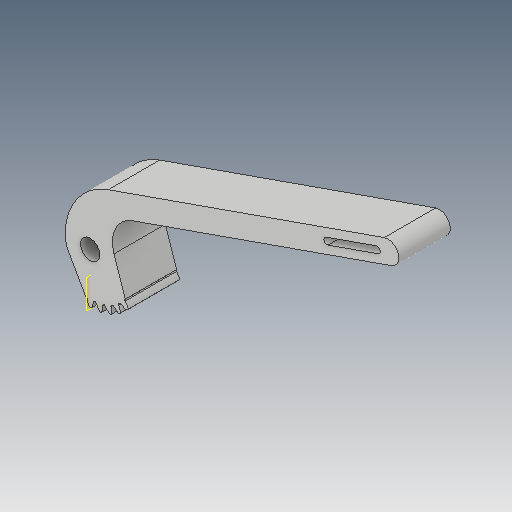
# Autodesk Inventor part: GripperLever_right_v2
Saved by Autodesk Inventor 2021.4 (Build 254397000, 397)
## iProperties
Created: 2022-04-22
Part Number: GripperLever_right_v2
Material: Generisch
Document SubType Name: Modeling
Designer: ALEX
Density: 1 g/cm^3
Appearance: Vorgabe
Mass: 2.14973 g
Surface Area: 19.5452 cm^2
Volume: 2.14973 cm^3
Di: 13,833 mm
GearThickness: 9,000 mm
Lever_Do: 8,000 mm
d: 15,000 mm
Author: ALEX
Autodesk Inventor part; units mm, degrees
ref_plane "YZ Plane" through (0, 0, 0) normal (1, 0, 0) x (0, 1, 0)
ref_plane "XZ Plane" through (0, 0, 0) normal (0, 1, 0) x (-1, 0, 0)
ref_plane "XY Plane" through (0, 0, 0) normal (0, 0, 1) x (1, 0, 0)
sketch "Skizze1" plane through (0, 0, 0) normal (0, 0, 1) x (1, 0, 0)
  circle A0 centre (0, 0) radius 6.9167 construction
  circle A1 centre (0, 0) radius 8 construction
  arc A2 (-0.4858, -7.0515) -> (-0.6563, -6.8855) centre (-0.6743, -7.0746) ccw
  arc A3 (-0.4858, -7.0515) -> (-0.1749, -7.9981) centre (2.0604, -6.7398) ccw
  line L0 (0, 0) -> (0.8362, -7.9562) construction
  line L1 (0, 0) -> (0, -8) construction
  arc A4 (-0.1749, -7.9981) -> (0.1749, -7.9981) centre (0, 0) ccw
  arc A5 (0.1749, -7.9981) -> (0.4858, -7.0515) centre (-2.0604, -6.7398) ccw
  arc A6 (0.6563, -6.8855) -> (0.4858, -7.0515) centre (0.6743, -7.0746) ccw
  arc A7 (0.6563, -6.8855) -> (0.723, -6.8788) centre (0, 0) ccw
  line L2 (0, 0) -> (0, -8) construction
  circle A8 centre (0, 0) radius 7.5 construction
  circle A9 centre (0, 0) radius 4
  circle A10 centre (0, 0) radius 1.55
  circle A11 centre (0, 0) radius 7.0477 construction
  line L3 (-0.3927, -7.4897) -> (2.0604, -6.7398) construction
  line L4 (0.3927, -7.4897) -> (-2.0604, -6.7398) construction
  line L5 (0, 0) -> (-0.723, -6.8788) construction
  arc A12 (-0.723, -6.8788) -> (-0.6563, -6.8855) centre (0, 0) ccw
  arc A13 (2.0735, -6.5985) -> (2.1374, -6.5781) centre (0, 0) ccw
  arc A14 (2.0735, -6.5985) -> (1.9412, -6.7964) centre (2.1305, -6.7798) ccw
  arc A15 (1.834, -7.7869) -> (1.9412, -6.7964) centre (-0.6141, -7.0209) ccw
  arc A16 (0.723, -6.8788) -> (0.7896, -6.8714) centre (0, 0) ccw
  arc A17 (1.4918, -7.8597) -> (1.834, -7.7869) centre (0, 0) ccw
  arc A18 (0.991, -6.9984) -> (0.7896, -6.8714) centre (0.8113, -7.0602) ccw
  arc A19 (0.991, -6.9984) -> (1.4918, -7.8597) centre (3.4166, -6.1641) ccw
  arc A20 (3.4001, -6.0232) -> (3.4583, -5.99) centre (0, 0) ccw
  arc A21 (3.4001, -6.0232) -> (3.3119, -6.2443) centre (3.4935, -6.1887) ccw
  arc A22 (3.4129, -7.2355) -> (3.3119, -6.2443) centre (0.8591, -6.9951) ccw
  arc A23 (2.1374, -6.5781) -> (2.201, -6.5571) centre (0, 0) ccw
  arc A24 (3.0933, -7.3778) -> (3.4129, -7.2355) centre (0, 0) ccw
  arc A25 (2.4243, -6.6395) -> (2.201, -6.5571) centre (2.2615, -6.7373) ccw
  arc A26 (2.4243, -6.6395) -> (3.0933, -7.3778) centre (4.6236, -5.3191) ccw
  arc A27 (4.5781, -5.1847) -> (4.6282, -5.1401) centre (0, 0) ccw
  arc A28 (4.5781, -5.1847) -> (4.5378, -5.4193) centre (4.7039, -5.3271) ccw
  arc A29 (4.8427, -6.3678) -> (4.5378, -5.4193) centre (2.2947, -6.6637) ccw
  arc A30 (3.4583, -5.99) -> (3.5162, -5.9562) centre (0, 0) ccw
  arc A31 (4.5596, -6.5734) -> (4.8427, -6.3678) centre (0, 0) ccw
  arc A32 (3.7518, -5.9903) -> (3.5162, -5.9562) centre (3.6128, -6.1198) ccw
  arc A33 (3.7518, -5.9903) -> (4.5596, -6.5734) centre (5.6284, -4.2415) ccw
  arc A34 (5.5561, -4.1195) -> (5.5957, -4.0655) centre (0, 0) ccw
  arc A35 (5.5561, -4.1195) -> (5.5653, -4.3574) centre (5.7087, -4.2327) ccw
  arc A36 (6.0608, -5.2218) -> (5.5653, -4.3574) centre (3.63, -6.041) ccw
  arc A37 (4.6282, -5.1401) -> (4.6777, -5.095) centre (0, 0) ccw
  arc A38 (5.8267, -5.4818) -> (6.0608, -5.2218) centre (0, 0) ccw
  arc A39 (4.9153, -5.0794) -> (4.6777, -5.095) centre (4.8062, -5.235) ccw
  arc A40 (4.9153, -5.0794) -> (5.8267, -5.4818) centre (6.3873, -2.9786) ccw
  line L6 (-0.723, -6.8788) -> (-3.4872, -1.9595)
  line L7 (5.5957, -4.0655) -> (3.7896, 1.2803)
  point P0 (2.4721, -7.6085)
  point P1 (1.9413, -7.2444)
  point P2 (1.6633, -7.8252)
  point P3 (1.6633, -7.8252)
  point P4 (1.1731, -7.4077)
  point P5 (4, -6.9282)
  point P6 (3.4051, -6.6825)
  point P7 (3.2539, -7.3084)
  point P8 (3.2539, -7.3084)
  point P9 (2.6876, -7.0019)
  point P10 (5.353, -5.9452)
  point P11 (4.72, -5.8285)
  point P12 (4.7023, -6.4721)
  point P13 (4.7023, -6.4721)
  point P14 (4.0846, -6.2901)
  point P15 (6.4721, -4.7023)
  point P16 (5.8287, -4.7198)
  point P17 (5.9452, -5.353)
  point P18 (5.9452, -5.353)
  point P19 (5.3032, -5.3034)
  point P20 (0.723, -6.8788)
  point P21 (2.1374, -6.5781)
  point P22 (3.4583, -5.99)
  point P23 (4.6282, -5.1401)
  point P24 (5.5957, -4.0655)
  dimension "d0" = 13.8333
  dimension "d1" = 16
  dimension "d2" = 0.19
  dimension "d6" = 0
  dimension "d9" = 15
  dimension "d10" = 0.7854
  dimension "Lever_Do" = 8
  dimension "d17" = 3.1
  dimension "d26" = 14.0954
  dimension "d74" = 12
  dimension "d75" = 6
  dimension "beta_circ" = 48
  constraints: 94 point on circle, 41 centre point, 16 end point, 8 coincident, 8 tangent, 3 concentric, 2 equal radius, 1 point on line, 1 vertical, 109 other
  measures "d0" diameter of A0
  measures "d1" diameter of A1
  measures "d2" radius of A2
  measures "d6" distance between parallel lines of L1 L2
  measures "d9" diameter of A8
  measures "d10" distance of L4.start L3.start
  measures "Lever_Do" diameter of A9
  measures "d17" diameter of A10
  measures "d26" diameter of A11
  measures "d74" angle of L0 L5
  measures "d75" angle of L5 L2
extrude "Extrusion1" add sketch "Skizze1" along normal blind 9
sketch "Skizze2" plane through (0, 0, 9) normal (0, 0, 1) x (1, 0, 0)
  line L0 (0, 0) -> (49.154, 0) construction
  arc A0 (3.7896, 1.2803) -> (-3.4872, -1.9595) centre (0, 0) ccw projected
  line L1 (48.5762, 25.6793) -> (49.7318, 22.3756)
  line L2 (49.3026, 23.6027) -> (2.1068, 7.0935) construction
  line L3 (0, 0) -> (1.1388, 3.8345) construction
  line L4 (49.154, 0) -> (49.154, 24.0275) construction
  circle A1 centre (0, 0) radius 4 construction
  line L5 (6.7484, 7.3399) -> (49.7318, 22.3756)
  line L6 (48.5762, 25.6793) -> (2.8793, 9.6944)
  circle A2 centre (0, 0) radius 8 construction
  arc A3 (2.8793, 9.6944) -> (-4, 0) centre (6.2704, 0) ccw
  arc A4 (6.7484, 7.3399) -> (3.7896, 1.2803) centre (8.3313, 2.8148) ccw
  circle A5 centre (0, 0) radius 1.55 projected
  line L7 (0, 0) -> (49.154, 17.1942) construction
  dimension "d39" = 19.28
  dimension "d70" = 8
  dimension "d72" = 50
  dimension "d96" = 6
  dimension "d97" = 1.3
  dimension "d98" = 3.5
  constraints: 16 end point, 6 point on circle, 5 point on line, 4 tangent, 3 centre point, 3 parallel, 2 coincident, 1 horizontal, 1 midpoint, 1 perpendicular, 1 vertical
  measures "d39" angle of L0 L2
  measures "d70" diameter of A1
  measures "d72" distance of L2.start L2.end
  measures "d96" distance between parallel lines of L7 L2
  measures "d97" distance between parallel lines of L5 L2
  measures "d98" distance between parallel lines of L6 L5
extrude "Extrusion2" add sketch "Skizze2" against normal up to surface (9 mm away) contours A0 A3 L6 L1 L5 A4
ref_plane "AdjustPlane_right" through (0, -8, 9) normal (1, 0, 0) x (0, 0, -1)
sketch "Sketch4" plane through (0, 0, 0) normal (0, 0, -1) x (-1, 0, 0)
  line L0 (-2.4788, -4.3156) -> (-2, -3) construction
  line L1 (-2, -3) -> (-0.4965, -3.5472) construction
  line L2 (-0.4965, -3.5472) -> (-0.9753, -4.8628) construction
  line L3 (-0.9753, -4.8628) -> (-2.4788, -4.3156) construction
  line L4 (0, 0) -> (0, -3) construction
  line L5 (0, -3) -> (-2, -3) construction
  line L6 (-0.6203, -3.595) -> (-0.7088, -3.8383)
  line L7 (-0.7088, -3.8383) -> (-1.4318, -4.0796)
  line L8 (-1.4318, -4.0796) -> (-1.51, -4.2944)
  line L9 (-1.51, -4.2944) -> (-0.9491, -4.4985)
  line L10 (-0.9491, -4.4985) -> (-1.0173, -4.6858)
  line L11 (-1.0173, -4.6858) -> (-2.4269, -4.1728)
  line L12 (-2.4269, -4.1728) -> (-2.2947, -3.8096)
  spline S0 degree 2 poles (-2.2947, -3.8096) (-2.2506, -3.6885) (-2.1649, -3.5347) (-2.0899, -3.4779) knots 0 0 0 1 2 2 2
  spline S1 degree 2 poles (-2.0899, -3.4779) (-2.0149, -3.4211) (-1.834, -3.3899) (-1.7232, -3.4302) knots 0 0 0 1 2 2 2
  spline S2 degree 2 poles (-1.7232, -3.4302) (-1.569, -3.4864) (-1.4174, -3.7201) (-1.4162, -3.8732) knots 0 0 0 1 2 2 2
  line L13 (-1.4162, -3.8732) -> (-0.6203, -3.595)
  spline S3 degree 2 poles (-1.7795, -3.631) (-1.8412, -3.6085) (-1.9518, -3.6174) (-1.9993, -3.6519) knots 0 0 0 1 2 2 2
  spline S4 degree 2 poles (-1.9993, -3.6519) (-2.0401, -3.6823) (-2.1004, -3.7806) (-2.1287, -3.8583) knots 0 0 0 1 2 2 2
  line L14 (-2.1287, -3.8583) -> (-2.1965, -4.0445)
  line L15 (-2.1965, -4.0445) -> (-1.6665, -4.2374)
  line L16 (-1.6665, -4.2374) -> (-1.6066, -4.0729)
  spline S5 degree 2 poles (-1.6066, -4.0729) (-1.5771, -3.9918) (-1.5587, -3.8523) (-1.587, -3.7916) knots 0 0 0 1 2 2 2
  spline S6 degree 2 poles (-1.587, -3.7916) (-1.6109, -3.7363) (-1.7064, -3.6576) (-1.7795, -3.631) knots 0 0 0 1 2 2 2
  dimension "d85" = 3
  dimension "d86" = 2
  dimension "d87" = 1.4
  dimension "d88" = 1.6
  dimension "d89" = 20
  constraints: 4 end point, 1 horizontal, 1 vertical, 2 other
  measures "d85" vertical distance of L4.start L0.end
  measures "d86" horizontal distance of L4.start L0.end
  measures "d87" distance of L0.start L0.end
  measures "d88" distance of L2.end L0.start
  measures "d89" angle of L2 L4
extrude "Extrusion3" cut sketch "Sketch4" against normal blind 0.5
thicken "Thicken1" operation add thickness 0.4 both sides no extend neighbours yes toward (0, 0, 1) faces at (19.4013, 14.2379, 0)
thicken "Thicken2" operation add thickness 0.4 both sides no extend neighbours yes toward (0, 0, -1) faces at (19.4013, 14.2379, 9)
delete faces "Delete Face1" heal yes whole lump no faces at (1.9773, -3.9919, 0) (2.1097, -3.8097, 0.25) (1.8199, -3.619, 0.25) (2.1513, -3.9204, 0.1667) (1.7336, -3.6501, 0.25) (1.5892, -4.0201, 0.25) (1.6465, -4.1826, 0.1667) (2.0198, -4.1088, 0.1667)
sketch "Sketch5" plane through (5.5957, -4.0655, 0.4) normal (0, 0, -1) x (-0.9473892, -0.320084, 0)
  line L0 (-50.2775, 10.9228) -> (-50.2401, 14.4226) construction
  line L1 (-50.2588, 12.6727) -> (-35.2596, 12.5124) construction
  line L2 (-46.709, 12.6347) -> (-38.2095, 12.544) construction
  line L3 (-46.7036, 13.1347) -> (-38.2041, 13.0439)
  line L4 (-38.2148, 12.044) -> (-46.7143, 12.1348)
  arc A0 (-46.7036, 13.1347) -> (-46.7143, 12.1348) centre (-46.709, 12.6347) ccw
  arc A1 (-38.2148, 12.044) -> (-38.2041, 13.0439) centre (-38.2095, 12.544) ccw
  point P0 (4, 5.6427)
  point P1 (-42.4592, 12.5894)
  dimension "d100" = 15
  dimension "d101" = 1
  dimension "d102" = 8.5
  dimension "d103" = 7.8
  constraints: 10 end point, 4 point on circle, 4 tangent, 2 centre point, 2 midpoint, 2 point on line, 1 parallel, 1 perpendicular
  measures "d100" distance of L1.start L1.end
  measures "d101" distance between parallel lines of L3 L4
  measures "d102" distance of L2.end L2.start
  measures "d103" distance from line of L0 point (-42.459, 12.589)
extrude "Extrusion4" cut sketch "Sketch5" against normal through all
fillet "Fillet1" radius 1.75 2 edges at (48.5762, 25.6793, 4.5) (49.7318, 22.3756, 4.5)
equation "\"d9\" = d"
equation "\"Gear_r\" = 0.38"
equation "\"Gear_R\" = 5.1303"
equation "\"modul\" = 0.5"
equation "\"Sp\" = 1.57008"
equation "\"TotalAngle\" = 48deg"
equation "\"alpha\" = 12deg"
equation "\"Do\" = 16"
equation "\"Di\" = 13.83333"
equation "\"p\" = 1.570796"
equation "\"delta_f\" = 0.19"
equation "\"Db\" = 14.09539"
equation "\"Kopfspiel\" = 0.58333"
equation "\"beta_circ_max\" = 60deg"
equation "\"d\" = 15"
